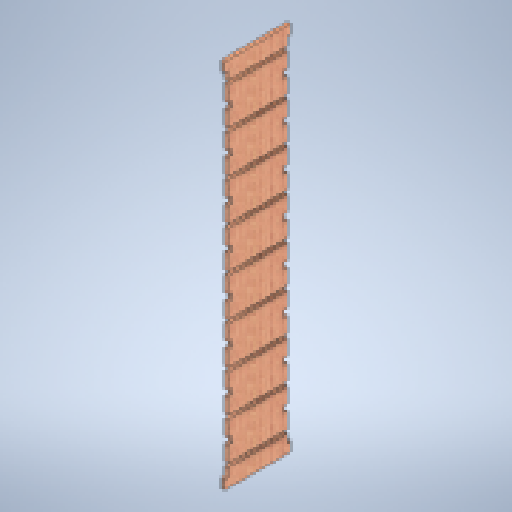
# Autodesk Inventor part: Separators
Saved by Autodesk Inventor 2024 (Build 280153000, 153)
## iProperties
Created: 2023-07-19
Part Number: Separators
Material: Generic
Document SubType Name: Modeling
Designer: Bruno
Density: 1 g/cm^3
Appearance: Default
Author: Bruno
Autodesk Inventor part; units mm, degrees
ref_plane "YZ Plane" through (0, 0, 0) normal (1, 0, 0) x (0, 1, 0)
ref_plane "XZ Plane" through (0, 0, 0) normal (0, 1, 0) x (-1, 0, 0)
ref_plane "XY Plane" through (0, 0, 0) normal (0, 0, 1) x (1, 0, 0)
sketch "Sketch1" plane through (0, 0, 0) normal (1, 0, 0) x (0, 1, 0)
  line L0 (0, 56) -> (0, 0)
  line L1 (15, 53) -> (15, 28)
  line L2 (15, 28) -> (16.55, 28)
  line L3 (16.55, 28) -> (18.1, 28)
  line L4 (18.1, 28) -> (18.1, 53)
  line L5 (18.1, 53) -> (31.55, 53)
  line L6 (31.55, 53) -> (31.55, 50)
  line L7 (31.55, 50) -> (36.55, 50)
  line L8 (36.55, 50) -> (36.55, 53)
  line L9 (36.55, 53) -> (50, 53)
  line L10 (50, 53) -> (50, 28)
  line L11 (50, 28) -> (51.55, 28)
  line L12 (16.55, 3) -> (31.55, 3)
  line L13 (31.55, 3) -> (31.55, 6)
  line L14 (31.55, 6) -> (36.55, 6)
  line L15 (36.55, 6) -> (36.55, 3)
  line L16 (36.55, 3) -> (51.55, 3)
  line L17 (51.55, 28) -> (53.1, 28)
  line L18 (53.1, 28) -> (53.1, 53)
  line L19 (53.1, 53) -> (66.55, 53)
  line L20 (66.55, 50) -> (71.55, 50)
  line L21 (66.55, 53) -> (66.55, 50)
  line L22 (71.55, 50) -> (71.55, 53)
  line L23 (71.55, 53) -> (85, 53)
  line L24 (85, 53) -> (85, 28)
  line L25 (85, 28) -> (86.55, 28)
  line L26 (71.55, 3) -> (86.55, 3)
  line L27 (66.55, 6) -> (71.55, 6)
  line L28 (71.55, 6) -> (71.55, 3)
  line L29 (66.55, 3) -> (66.55, 6)
  line L30 (51.55, 3) -> (66.55, 3)
  line L31 (86.55, 28) -> (88.1, 28)
  line L32 (88.1, 28) -> (88.1, 53)
  line L33 (88.1, 53) -> (101.55, 53)
  line L34 (101.55, 50) -> (106.55, 50)
  line L35 (101.55, 53) -> (101.55, 50)
  line L36 (106.55, 50) -> (106.55, 53)
  line L37 (106.55, 53) -> (120, 53)
  line L38 (120, 53) -> (120, 28)
  line L39 (120, 28) -> (121.55, 28)
  line L40 (106.55, 3) -> (121.55, 3)
  line L41 (101.55, 6) -> (106.55, 6)
  line L42 (106.55, 6) -> (106.55, 3)
  line L43 (101.55, 3) -> (101.55, 6)
  line L44 (86.55, 3) -> (101.55, 3)
  line L45 (121.55, 28) -> (123.1, 28)
  line L46 (123.1, 28) -> (123.1, 53)
  line L47 (123.1, 53) -> (136.55, 53)
  line L48 (136.55, 50) -> (141.55, 50)
  line L49 (136.55, 53) -> (136.55, 50)
  line L50 (141.55, 50) -> (141.55, 53)
  line L51 (141.55, 53) -> (155, 53)
  line L52 (155, 53) -> (155, 28)
  line L53 (155, 28) -> (156.55, 28)
  line L54 (141.55, 3) -> (156.55, 3)
  line L55 (136.55, 6) -> (141.55, 6)
  line L56 (141.55, 6) -> (141.55, 3)
  line L57 (136.55, 3) -> (136.55, 6)
  line L58 (121.55, 3) -> (136.55, 3)
  line L59 (156.55, 28) -> (158.1, 28)
  line L60 (158.1, 28) -> (158.1, 53)
  line L61 (158.1, 53) -> (171.55, 53)
  line L62 (171.55, 50) -> (176.55, 50)
  line L63 (171.55, 53) -> (171.55, 50)
  line L64 (176.55, 50) -> (176.55, 53)
  line L65 (176.55, 53) -> (190, 53)
  line L66 (190, 53) -> (190, 28)
  line L67 (190, 28) -> (191.55, 28)
  line L68 (176.55, 3) -> (191.55, 3)
  line L69 (171.55, 6) -> (176.55, 6)
  line L70 (176.55, 6) -> (176.55, 3)
  line L71 (171.55, 3) -> (171.55, 6)
  line L72 (156.55, 3) -> (171.55, 3)
  line L73 (191.55, 28) -> (193.1, 28)
  line L74 (193.1, 28) -> (193.1, 53)
  line L75 (193.1, 53) -> (206.55, 53)
  line L76 (206.55, 50) -> (211.55, 50)
  line L77 (206.55, 53) -> (206.55, 50)
  line L78 (211.55, 50) -> (211.55, 53)
  line L79 (211.55, 53) -> (225, 53)
  line L80 (225, 53) -> (225, 28)
  line L81 (225, 28) -> (226.55, 28)
  line L82 (211.55, 3) -> (226.55, 3)
  line L83 (206.55, 6) -> (211.55, 6)
  line L84 (211.55, 6) -> (211.55, 3)
  line L85 (206.55, 3) -> (206.55, 6)
  line L86 (191.55, 3) -> (206.55, 3)
  line L87 (226.55, 28) -> (228.1, 28)
  line L88 (228.1, 28) -> (228.1, 53)
  line L89 (228.1, 53) -> (241.55, 53)
  line L90 (241.55, 50) -> (246.55, 50)
  line L91 (241.55, 53) -> (241.55, 50)
  line L92 (246.55, 50) -> (246.55, 53)
  line L93 (246.55, 53) -> (260, 53)
  line L94 (260, 53) -> (260, 28)
  line L95 (260, 28) -> (261.55, 28)
  line L96 (246.55, 3) -> (261.55, 3)
  line L97 (241.55, 6) -> (246.55, 6)
  line L98 (246.55, 6) -> (246.55, 3)
  line L99 (241.55, 3) -> (241.55, 6)
  line L100 (226.55, 3) -> (241.55, 3)
  line L101 (261.55, 28) -> (263.1, 28)
  line L102 (263.1, 28) -> (263.1, 53)
  line L103 (263.1, 53) -> (276.55, 53)
  line L104 (276.55, 50) -> (281.55, 50)
  line L105 (276.55, 53) -> (276.55, 50)
  line L106 (281.55, 50) -> (281.55, 53)
  line L107 (281.55, 53) -> (295, 53)
  line L108 (295, 53) -> (295, 28)
  line L109 (295, 28) -> (296.55, 28)
  line L110 (281.55, 3) -> (296.55, 3)
  line L111 (276.55, 6) -> (281.55, 6)
  line L112 (281.55, 6) -> (281.55, 3)
  line L113 (276.55, 3) -> (276.55, 6)
  line L114 (261.55, 3) -> (276.55, 3)
  line L115 (156.55, 3) -> (156.55, 28) construction
  line L116 (15, 3) -> (16.55, 3)
  line L117 (0, 56) -> (8, 56)
  line L118 (8, 56) -> (8, 53)
  line L119 (8, 53) -> (15, 53)
  line L120 (0, 0) -> (8, 0)
  line L121 (8, 0) -> (8, 3)
  line L122 (8, 3) -> (16.55, 3)
  line L123 (313.1, 56) -> (313.1, 0)
  line L124 (298.1, 53) -> (298.1, 28)
  line L125 (298.1, 28) -> (296.55, 28)
  line L126 (298.1, 3) -> (296.55, 3)
  line L127 (313.1, 56) -> (305.1, 56)
  line L128 (305.1, 56) -> (305.1, 53)
  line L129 (305.1, 53) -> (298.1, 53)
  line L130 (313.1, 0) -> (305.1, 0)
  line L131 (305.1, 0) -> (305.1, 3)
  line L132 (305.1, 3) -> (296.55, 3)
  point P0 (15.775, 28)
  point P1 (297.325, 28)
  dimension "d36" = 1.55
  dimension "d37" = 1.55
  dimension "d39" = 5
  dimension "d41" = 1.55
  dimension "d42" = 35
  dimension "d43" = 5
  dimension "d45" = 3
  dimension "d46" = 35
  dimension "d51" = 35
  dimension "d61" = 25
  dimension "d62" = 50
  dimension "d63" = 3
  dimension "d66" = 3
  dimension "d67" = 8
  dimension "d68" = 7
  constraints: 266 end point, 48 point on line, 13 perpendicular, 11 symmetric about line, 6 horizontal, 5 collinear, 3 vertical alignment, 2 coincident, 2 vertical, 1 horizontal alignment, 1 midpoint, 1 parallel, 209 other
  measures "d36" distance of L1.end L2.end
  measures "d37" distance of L2.end L3.end
  measures "d39" distance of L6.end L7.end
  measures "d41" distance of L10.end L11.end
  measures "d42" distance of L11.end L2.end
  measures "d43" distance of L13.end L14.end
  measures "d45" distance of L12.end L13.end
  measures "d46" distance of L12.start L16.end
  measures "d51" distance of L3.end L17.end
  measures "d61" distance from line of L5 point (15.775, 28)
  measures "d62" distance between parallel lines of L12 L5
  measures "d63" distance of L7.end L8.end
  measures "d66" distance between parallel lines of L117 L5
  measures "d67" distance of L0.start L117.end
  measures "d68" distance of L118.end L1.start
extrude "Extrusion1" add sketch "Sketch1" along normal blind 3
body "Solid1"
